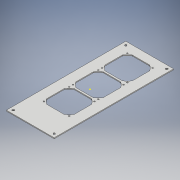
# Autodesk Inventor part: top_panel2
Saved by Autodesk Inventor 2018 (Build 220112000, 112)
## iProperties
Created: 2021-05-16
Part Number: top_panel2
Material: Generic
Document SubType Name: Modeling
Designer: gisen
Density: 1 g/cm^3
Appearance: Default
Author: gisen
Autodesk Inventor part; units mm, degrees
ref_plane "YZ Plane" through (0, 0, 0) normal (1, 0, 0) x (0, 1, 0)
ref_plane "XZ Plane" through (0, 0, 0) normal (0, 1, 0) x (-1, 0, 0)
ref_plane "XY Plane" through (0, 0, 0) normal (0, 0, 1) x (1, 0, 0)
sketch "Sketch1" plane through (0, 0, 0) normal (0, 0, 1) x (1, 0, 0)
  line L0 (-78, 195) -> (78, 195)
  line L1 (78, 195) -> (78, -195)
  line L2 (78, -195) -> (-78, -195)
  line L3 (-78, -195) -> (-78, 195)
  line L4 (-78, 195) -> (78, -195) construction
  line L5 (78, 195) -> (-78, -195) construction
  point P0 (0, 0)
  dimension "d1" = 156
  dimension "d2" = 390
  constraints: 12 end point, 2 midpoint, 2 parallel, 1 horizontal, 1 perpendicular
  measures "d1" distance of L0.start L0.end
  measures "d2" distance of L0.end L1.end
extrude "Extrusion1" add sketch "Sketch1" along normal blind 3
sketch "Sketch2" plane through (0, 0, 3) normal (0, 0, 1) x (1, 0, 0)
  line L0 (-78, -195) -> (78, -195) projected
  line L1 (-78, 195) -> (-78, -195) projected
  arc A0 (-64.4298, -185.2577) -> (-68.2577, -181.4298) centre (-66, -183) ccw
  arc A1 (-69.8472, -183.7153) -> (-66.7153, -186.8472) centre (-68, -185) ccw
  line L2 (-66.7153, -186.8472) -> (-64.4298, -185.2577)
  line L3 (-69.8472, -183.7153) -> (-68.2577, -181.4298)
  line L4 (0, 16.0888) -> (0, -25.3045)
  line L5 (-19.6832, 0) -> (22.709, 0)
  arc A2 (68.2577, -181.4298) -> (64.4298, -185.2577) centre (66, -183) ccw
  arc A3 (66.7153, -186.8472) -> (69.8472, -183.7153) centre (68, -185) ccw
  line L6 (66.7153, -186.8472) -> (64.4298, -185.2577)
  line L7 (69.8472, -183.7153) -> (68.2577, -181.4298)
  arc A4 (-68.2577, 181.4298) -> (-64.4298, 185.2577) centre (-66, 183) ccw
  arc A5 (-66.7153, 186.8472) -> (-69.8472, 183.7153) centre (-68, 185) ccw
  line L8 (-66.7153, 186.8472) -> (-64.4298, 185.2577)
  line L9 (-69.8472, 183.7153) -> (-68.2577, 181.4298)
  arc A6 (64.4298, 185.2577) -> (68.2577, 181.4298) centre (66, 183) ccw
  arc A7 (69.8472, 183.7153) -> (66.7153, 186.8472) centre (68, 185) ccw
  line L10 (66.7153, 186.8472) -> (64.4298, 185.2577)
  line L11 (69.8472, 183.7153) -> (68.2577, 181.4298)
  point P0 (0, 0)
  dimension "d11" = 12
  dimension "d12" = 10
  dimension "d13" = 12
  dimension "d14" = 10
  dimension "d15" = 5.5
  dimension "d16" = 4.5
  constraints: 24 symmetric about line, 20 end point, 16 point on circle, 8 centre point, 8 coincident, 4 tangent, 1 horizontal, 1 vertical, 6 other
  measures "d11" distance from line of L0 point (-66, -183)
  measures "d12" distance from line of L0 point (-68, -185)
  measures "d13" distance from line of L1 point (-66, -183)
  measures "d14" distance from line of L1 point (-68, -185)
  measures "d15" diameter of A0
  measures "d16" diameter of A1
extrude "Extrusion2" cut sketch "Sketch2" against normal up to surface (3 mm away)
sketch "Sketch3" plane through (0, 0, 3) normal (0, 0, 1) x (1, 0, 0)
  line L0 (78, 195) -> (-78, 195) projected
  line L1 (28.4765, 166.7) -> (-28.4765, 166.7)
  circle A0 centre (-41.25, 163.25) radius 2.25
  line L2 (-28.4765, 77.3) -> (28.4765, 77.3)
  circle A1 centre (-41.25, 80.75) radius 2.25
  circle A2 centre (41.25, 80.75) radius 2.25
  circle A3 centre (41.25, 163.25) radius 2.25
  line L3 (44.7, 93.5235) -> (44.7, 150.4765)
  line L4 (-44.7, 150.4765) -> (-44.7, 93.5235)
  arc A4 (28.4765, 77.3) -> (44.7, 93.5235) centre (0, 122) ccw
  arc A5 (44.7, 150.4765) -> (28.4765, 166.7) centre (0, 122) ccw
  arc A6 (-28.4765, 166.7) -> (-44.7, 150.4765) centre (0, 122) ccw
  arc A7 (-44.7, 93.5235) -> (-28.4765, 77.3) centre (0, 122) ccw
  line L5 (28.4765, -17.7) -> (-28.4765, -17.7)
  circle A8 centre (-41.25, -14.25) radius 2.25
  line L6 (-28.4765, 71.7) -> (28.4765, 71.7)
  circle A9 centre (-41.25, 68.25) radius 2.25
  circle A10 centre (41.25, 68.25) radius 2.25
  circle A11 centre (41.25, -14.25) radius 2.25
  line L7 (44.7, 55.4765) -> (44.7, -1.4765)
  line L8 (-44.7, -1.4765) -> (-44.7, 55.4765)
  arc A12 (44.7, 55.4765) -> (28.4765, 71.7) centre (0, 27) ccw
  arc A13 (28.4765, -17.7) -> (44.7, -1.4765) centre (0, 27) ccw
  arc A14 (-44.7, -1.4765) -> (-28.4765, -17.7) centre (0, 27) ccw
  arc A15 (-28.4765, 71.7) -> (-44.7, 55.4765) centre (0, 27) ccw
  circle A16 centre (41.25, -109.25) radius 2.25
  arc A17 (28.4765, -112.7) -> (44.7, -96.4765) centre (0, -68) ccw
  line L9 (44.7, -96.4765) -> (44.7, -39.5235)
  line L10 (-28.4765, -112.7) -> (28.4765, -112.7)
  circle A18 centre (41.25, -26.75) radius 2.25
  arc A19 (44.7, -39.5235) -> (28.4765, -23.3) centre (0, -68) ccw
  circle A20 centre (-41.25, -109.25) radius 2.25
  arc A21 (-44.7, -96.4765) -> (-28.4765, -112.7) centre (0, -68) ccw
  line L11 (-44.7, -39.5235) -> (-44.7, -96.4765)
  line L12 (28.4765, -23.3) -> (-28.4765, -23.3)
  circle A22 centre (-41.25, -26.75) radius 2.25
  arc A23 (-28.4765, -23.3) -> (-44.7, -39.5235) centre (0, -68) ccw
  point P0 (0, 0)
  dimension "d20" = 73
  dimension "d21" = 41.25
  dimension "d22" = 41.25
  dimension "d24" = 44.7
  dimension "d25" = 4.5
  dimension "d27" = 44.7
  dimension "d31" = 360
  constraints: 24 centre point, 24 end point, 24 point on circle, 13 coincident, 2 horizontal, 1 perpendicular, 1 vertical, 13 other
  measures "d20" distance from line of point (0, 122) L0
  measures "d21" horizontal distance of point (0, 122) point (-41.25, 163.25)
  measures "d22" horizontal distance of point (0, 122) point (-41.25, 163.25)
  measures "d24" distance from line of point (0, 122) L1
  measures "d25" diameter of A0
  measures "d27" distance from line of point (0, 122) L2
extrude "Extrusion3" cut sketch "Sketch3" against normal up to surface (3 mm away)
sketch "Sketch4" plane through (0, 0, 3) normal (0, 0, 1) x (1, 0, 0)
  point P0 (0, 0)
equation "\"d13\" = d11"
equation "\"d14\" = d12"
equation "\"d27\" = d24"
equation "\"d26\" = d24"
equation "\"d28\" = d26"
body "Solid1"
